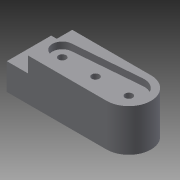
# Autodesk Inventor part: servo_clip1
Saved by Autodesk Inventor 2015 (Build 190159000, 159)
## iProperties
Created: 2017-12-02
Part Number: servo_clip1
Material: Generic
Document SubType Name: Modeling
Designer: Anshul
Density: 1 g/cm^3
Appearance: Default
Author: Anshul
Autodesk Inventor part; units mm, degrees
ref_plane "YZ Plane" through (0, 0, 0) normal (1, 0, 0) x (0, 1, 0)
ref_plane "XZ Plane" through (0, 0, 0) normal (0, 1, 0) x (-1, 0, 0)
ref_plane "XY Plane" through (0, 0, 0) normal (0, 0, 1) x (1, 0, 0)
sketch "Sketch1" plane through (0, 0, 0) normal (0, 1, 0) x (-1, 0, 0)
  line L0 (0, 0) -> (0, -16)
  line L1 (0, 0) -> (0, -30)
  line L2 (0, -16) -> (0, -20)
  line L3 (0, -16) -> (50, -16)
  line L4 (50, -16) -> (50, 0)
  line L5 (50, 0) -> (0, 0)
  line L6 (50, -20) -> (50, -16)
  arc A0 (0.5833, -23.0243) -> (0.5833, -36.9757) centre (0, -30) ccw
  line L7 (0, -30) -> (30, -30)
  circle A1 centre (30, -30) radius 4.5
  line L8 (30.375, -25.5157) -> (0.5833, -23.0243)
  line L9 (30.375, -34.4843) -> (0.5833, -36.9757)
  line L10 (0, -40) -> (45, -40)
  line L11 (45, -40) -> (45, -20)
  line L12 (45, -20) -> (0, -20)
  circle A2 centre (30, -30) radius 1.7
  circle A3 centre (15, -30) radius 1.7
  line L13 (45, -30) -> (40, -30)
  circle A4 centre (40, -30) radius 1.7
  circle A5 centre (0, -30) radius 3.15
  circle A6 centre (0, -30) radius 1.7
  line L14 (45, -20) -> (0, -20)
  line L15 (45, -20) -> (35.5, -20)
  line L16 (35.5, -20) -> (35.5, -40)
  arc A7 (0, -20) -> (0, -40) centre (0, -30) ccw
  dimension "d0" = 16
  dimension "d1" = 30
  dimension "d2" = 4
  dimension "d3" = 50
  dimension "d4" = 50
  dimension "d22" = 14
  dimension "d23" = 30
  dimension "d24" = 9
  dimension "d26" = 45
  dimension "d29" = 3.4
  dimension "d30" = 3.4
  dimension "d31" = 5
  dimension "d32" = 3.4
  dimension "d34" = 6.3
  dimension "d35" = 3.4
  dimension "d36" = 9.5
  constraints: 34 end point, 8 centre point, 6 coincident, 6 point on circle, 5 perpendicular, 4 point on line, 4 tangent, 3 horizontal, 2 midpoint, 2 vertical, 1 collinear
  measures "d0" distance of L0.start L0.end
  measures "d1" distance of L0.start L1.end
  measures "d2" distance of L0.end L2.end
  measures "d3" distance of L0.end L3.end
  measures "d4" distance of L2.end L6.start
  measures "d22" diameter of A0
  measures "d23" distance of L7.start L7.end
  measures "d24" diameter of A1
  measures "d26" distance of L10.start L10.end
  measures "d29" diameter of A2
  measures "d30" diameter of A3
  measures "d31" distance of L13.start L13.end
  measures "d32" diameter of A4
  measures "d34" diameter of A5
  measures "d35" diameter of A6
  measures "d36" distance of L11.end L15.end
extrude "Extrusion4" add sketch "Sketch1" along normal blind 16 contours A0 L8 A1 L7 A3 A5 L1 | L1 A5 L7 A3 A1 L9 A0 | A5 L7 A6 L1 | L1 A6 L7 A5 | A1
extrude "Extrusion5" add sketch "Sketch1" along normal blind 19 contours L12 L16 L10 A7
extrude "Extrusion6" add sketch "Sketch1" along normal blind 12 contours L12 L11 L10 L16
extrude "Extrusion7" cut sketch "Sketch1" along normal blind 5 contours A5 L7 A6 L1 | L1 A6 L7 A5
body "Solid2"
